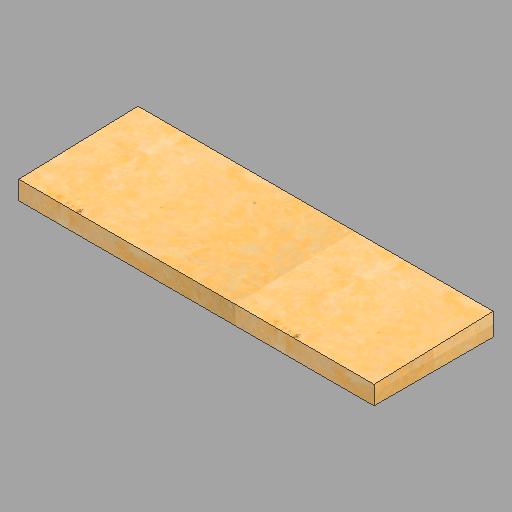
# Autodesk Inventor part: Coping - 4
Saved by Autodesk Inventor 2023 (Build 270158030, 158C)
## iProperties
RuleStatus: InUse
Created: 2022-06-13
Part Number: Coping - 4
Material: Granite, Cut, Polished
Document SubType Name: Modeling
Designer: awelt
Mass: 92822.6 g
Surface Area: 12130.2 cm^2
Volume: 34378.7 cm^3
Density: 2.7 g/cm^3
Appearance: Amber Select
AfterDocSave0: Convert in3 volume to ft3
in3 to ft3: 0.0
TEST: 0.001
Author: awelt
Autodesk Inventor part; units mm, degrees
ref_plane "YZ Plane" through (0, 0, 0) normal (1, 0, 0) x (0, 1, 0)
ref_plane "XZ Plane" through (0, 0, 0) normal (0, 1, 0) x (-1, 0, 0)
ref_plane "XY Plane" through (0, 0, 0) normal (0, 0, 1) x (1, 0, 0)
sketch "Sketch1" plane through (0, 0, 0) normal (1, 0, 0) x (0, 1, 0)
  line L0 (0, 0) -> (76.2, 0)
  line L1 (0, 0) -> (0, 406.4)
  line L2 (0, 406.4) -> (63.5, 406.4)
  line L3 (63.5, 406.4) -> (76.2, 0)
  dimension "d0" = 76.2
  dimension "d1" = 406.4
  dimension "d2" = 63.5
  constraints: 8 end point, 1 horizontal, 1 perpendicular, 1 vertical
  measures "d0" distance of L0.start L0.end
  measures "d1" distance of L0.start L1.end
  measures "d2" distance of L1.end L2.end
extrude "Extrusion1" add sketch "Sketch1" along normal blind 1211.2625
sketch "Sketch2" plane through (0, 0, 0) normal (0, -1, 0) x (1, 0, 0)
  line L0 (0, 406.4) -> (1211.2625, 406.4) projected
  line L1 (1211.2625, 406.4) -> (1211.2625, 0) projected
  line L2 (0, 406.4) -> (0, 0) projected
  line L3 (1211.2625, 0) -> (1211.2625, 406.4) construction
  line L4 (1211.2625, 219.075) -> (0, 219.075) construction
  line L5 (0, 406.4) -> (1211.2625, 406.4) construction
  line L6 (1012.0312, 406.4) -> (1012.0312, 0) construction
  line L7 (0, 0) -> (1211.2625, 0) construction
  line L8 (199.2312, 406.4) -> (199.2312, 0) construction
  line L9 (605.6313, 0) -> (605.6313, 406.4) construction
  circle A0 centre (1012.0312, 219.075) radius 4.7625
  circle A1 centre (199.2312, 219.075) radius 4.7625
  dimension "d5" = 187.325
  dimension "d6" = 812.8
  dimension "d7" = 9.525
  dimension "d8" = 9.525
  constraints: 10 point on line, 8 end point, 2 centre point, 2 coincident, 2 midpoint, 2 perpendicular, 1 symmetric about line, 1 vertical
  measures "d5" distance between parallel lines of L4 L0
  measures "d6" distance between parallel lines of L8 L6
  measures "d7" diameter of A0
  measures "d8" diameter of A1
extrude "Extrusion2" cut sketch "Sketch2" against normal blind 38.1
equation "\"d8\" = d7"
body "Solid1"
